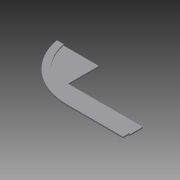
# Autodesk Inventor part: Arm-X25-Left-Back
Saved by Autodesk Inventor 2015 (Build 190159000, 159)
## iProperties
Created: 2018-07-01
Part Number: Arm-X25-Left-Back
Material: Generic
Document SubType Name: Modeling
Designer: Equipments
Density: 1 g/cm^3
Appearance: Default
Author: Equipments
Autodesk Inventor part; units mm, degrees
ref_plane "YZ Plane" through (0, 0, 0) normal (1, 0, 0) x (0, 1, 0)
ref_plane "XZ Plane" through (0, 0, 0) normal (0, 1, 0) x (-1, 0, 0)
ref_plane "XY Plane" through (0, 0, 0) normal (0, 0, 1) x (1, 0, 0)
sketch "Sketch2" plane through (0, 0, 0) normal (0, 0, 1) x (1, 0, 0)
  line L0 (0, 0) -> (170, 0)
  line L1 (0, 70) -> (0, 0)
  line L2 (170, 0) -> (170, -30)
  line L3 (170, -30) -> (-80, -30)
  line L4 (-80, 70) -> (0, 70)
  line L5 (-80, 70) -> (-80, -30)
  dimension "d2" = 30
  dimension "d5" = 70
  dimension "d9" = 80
  dimension "d10" = 250
  constraints: 12 end point, 3 perpendicular, 2 vertical, 1 horizontal
  measures "d2" distance of L0.end L2.end
  measures "d5" distance of L1.start L0.start
  measures "d9" distance of L4.start L1.start
  measures "d10" distance of L2.end L3.end
extrude "Extrusion1" add sketch "Sketch2" along normal blind 3
fillet "Fillet1" radius 125 1 edges at (-80, -30, 1.5)
sketch "Sketch3" plane through (0, 0, 3) normal (0, 0, 1) x (1, 0, 0)
  arc A0 (-80, 70) -> (42.4745, -30) centre (42.4745, 95) ccw projected
  arc A1 (-95.2753, 70) -> (42.4745, -45) centre (42.4745, 95) ccw
  line L0 (170, -30) -> (170, -45)
  line L1 (-80, 70) -> (-95.2753, 70)
  line L2 (0, 70) -> (-80, 70) projected
  line L3 (170, -45) -> (42.4745, -45)
  line L4 (42.4745, -30) -> (170, -30) projected
  arc A2 (-80, 70) -> (42.4745, -30) centre (42.4745, 95) ccw
  line L5 (170, -30) -> (42.4745, -30)
  line L6 (170, -30) -> (170, 0) projected
  point P0 (0, 0)
  dimension "d12" = 280
  constraints: 9 end point, 4 point on circle, 2 centre point, 2 coincident, 2 tangent, 1 collinear, 1 concentric, 1 parallel, 1 perpendicular, 1 vertical
  measures "d12" diameter of A1
extrude "Extrusion2" add sketch "Sketch3" along normal blind 3
body "Solid1"
